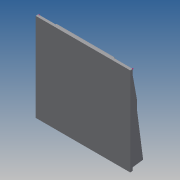
# Autodesk Inventor part: Bottom
Saved by Autodesk Inventor 2019 (Build 230136000, 136)
## iProperties
Created: 2022-10-28
Part Number: Bottom
Material: Generisch
Document SubType Name: Modeling
Designer: Dominik Schmidt
Density: 1 g/cm^3
Appearance: Vorgabe
Author: Dominik Schmidt
Autodesk Inventor part; units mm, degrees
ref_plane "YZ Plane" through (0, 0, 0) normal (1, 0, 0) x (0, 1, 0)
ref_plane "XZ Plane" through (0, 0, 0) normal (0, 1, 0) x (-1, 0, 0)
ref_plane "XY Plane" through (0, 0, 0) normal (0, 0, 1) x (1, 0, 0)
sketch "Skizze1" plane through (0, 0, 0) normal (0, 0, 1) x (1, 0, 0)
  line L0 (0, 0) -> (0, -76.0602) projected
  line L1 (0, -76.0602) -> (-35.95, -76.0602) projected
  line L2 (-45.45, -76.0602) -> (-81.4, -76.0602) projected
  line L3 (-81.4, -76.0602) -> (-81.4, 0) projected
  line L4 (-81.4, 0) -> (0, 0) projected
  line L5 (0, -76.0602) -> (-81.4, -76.0602)
  line L6 (-81.4, -76.0602) -> (-81.4, 0)
  line L7 (-81.4, 0) -> (0, 0)
  line L8 (0, 0) -> (0, -76.0602)
  constraints: 8 end point, 2 parallel, 1 horizontal, 1 perpendicular
extrude "Extrusion1" add sketch "Skizze1" along normal blind 2
sketch "Skizze2" plane through (0, 0, 0) normal (0, 0, -1) x (-1, 0, 0)
  point P0 (0, 0)
sketch "Skizze3" plane through (0, 0, 0) normal (0, 0, -1) x (-1, 0, 0)
  line L0 (35.95, -74.8497) -> (1.2, -74.8497) projected
  line L1 (80.2, -74.8497) -> (45.45, -74.8497) projected
  line L2 (49.95, -74.8497) -> (31.45, -74.8497)
  line L3 (31.45, -74.8497) -> (31.45, -50.3497)
  line L4 (31.45, -50.3497) -> (49.95, -50.3497)
  line L5 (49.95, -50.3497) -> (49.95, -74.8497)
  line L6 (81.4, 0) -> (81.4, -76.0602) projected
  line L7 (31.45, -50.3497) -> (29.45, -50.3497)
  line L8 (29.45, -50.3497) -> (29.45, -53.3497)
  line L9 (29.45, -53.3497) -> (31.45, -53.3497)
  line L10 (31.45, -53.3497) -> (31.45, -50.3497)
  line L11 (49.95, -50.3497) -> (51.95, -50.3497)
  line L12 (51.95, -50.3497) -> (51.95, -53.3497)
  line L13 (51.95, -53.3497) -> (49.95, -53.3497)
  line L14 (49.95, -53.3497) -> (49.95, -50.3497)
  line L15 (31.45, -50.3497) -> (34.45, -50.3497)
  line L16 (34.45, -50.3497) -> (34.45, -48.3497)
  line L17 (34.45, -48.3497) -> (31.45, -48.3497)
  line L18 (31.45, -48.3497) -> (31.45, -50.3497)
  line L19 (49.95, -50.3497) -> (46.95, -50.3497)
  line L20 (46.95, -50.3497) -> (46.95, -48.3497)
  line L21 (46.95, -48.3497) -> (49.95, -48.3497)
  line L22 (49.95, -48.3497) -> (49.95, -50.3497)
  line L23 (51.95, -50.3497) -> (49.95, -50.3497)
  line L24 (49.95, -50.3497) -> (49.95, -48.3497)
  line L25 (49.95, -48.3497) -> (51.95, -48.3497)
  line L26 (51.95, -48.3497) -> (51.95, -50.3497)
  line L27 (31.45, -50.3497) -> (29.45, -50.3497)
  line L28 (29.45, -50.3497) -> (29.45, -48.3497)
  line L29 (29.45, -48.3497) -> (31.45, -48.3497)
  line L30 (31.45, -48.3497) -> (31.45, -50.3497)
  point P0 (0, 0)
  dimension "d2" = 18.5
  dimension "d3" = 24.5
  dimension "d4" = 31.45
  dimension "d5" = 2
  dimension "d6" = 3
  dimension "d7" = 2
  dimension "d8" = 3
  dimension "d9" = 3
  dimension "d10" = 2
  dimension "d11" = 3
  dimension "d12" = 2
  constraints: 56 end point, 14 parallel, 7 horizontal, 7 perpendicular, 2 point on line
  measures "d2" distance of L3.end L4.end
  measures "d3" distance of L2.end L3.end
  measures "d4" distance between parallel lines of L6 L5
  measures "d5" distance of L9.end L8.end
  measures "d6" distance of L8.end L7.end
  measures "d7" distance of L12.end L13.end
  measures "d8" distance of L11.end L12.end
  measures "d9" distance of L17.end L16.end
  measures "d10" distance of L16.end L15.end
  measures "d11" distance of L20.end L21.end
  measures "d12" distance of L19.end L20.end
extrude "Extrusion2" add sketch "Skizze3" along normal blind 5 contours L9 L8 L7 L3 | L18 L17 L16 L4 | L7 L28 L29 L18 | L5 L11 L12 L13 | L22 L25 L26 L11 | L4 L20 L21 L22
sketch "Skizze4" plane through (-29.45, -53.3497, 0) normal (1, 0, 0) x (0, 0, -1)
  line L0 (9.1283, -19.2806) -> (0.7139, 44.1639) projected
  line L1 (0, -22.7105) -> (0, 53.3497) projected
  line L2 (5.629, 7.1044) -> (6.7525, -1.3669)
  line L3 (6.7525, -1.3669) -> (5.2084, -1.5716)
  line L4 (5.2084, -1.5716) -> (4.0849, 6.8996)
  line L5 (4.0849, 6.8996) -> (5.629, 7.1044)
  line L6 (5.629, 7.1044) -> (6.7525, -1.3669)
  line L7 (6.7525, -1.3669) -> (5.2084, -1.5716)
  line L8 (5.2084, -1.5716) -> (4.0849, 6.8996)
  line L9 (4.0849, 6.8996) -> (5.629, 7.1044)
  line L10 (5.629, 7.1044) -> (6.7525, -1.3669)
  line L11 (6.7525, -1.3669) -> (4.7916, -1.6269)
  line L12 (4.7916, -1.6269) -> (3.6681, 6.8444)
  line L13 (3.6681, 6.8444) -> (5.629, 7.1044)
  dimension "d17" = 1.978
  constraints: 24 end point, 6 parallel, 3 perpendicular, 2 collinear, 2 point on line
  measures "d17" distance of L2.end L11.end
extrude "Extrusion4" cut sketch "Skizze4" against normal blind 38.25
sketch "Skizze5" plane through (-51.95, -53.3497, 0) normal (-1, 0, 0) x (0, 0, 1)
  line L0 (-3.9127, 5) -> (-4.5759, 0) projected
  line L1 (0, 0) -> (-4.5759, 0) projected
  line L2 (0, 5) -> (0, 0) projected
  line L3 (0, 5) -> (-3.9127, 5) projected
  point P0 (0, 53.3497)
extrude "Extrusion5" add sketch "Skizze5" along normal blind 20
sketch "Skizze6" plane through (-71.95, -53.3497, 0) normal (-1, 0, 0) x (0, 0, 1)
  line L0 (-6.4924, -14.4505) -> (-0.5768, 30.1527)
  line L1 (-4.5759, 0) -> (-4.178, 3) projected
  line L2 (-0.5768, 30.1527) -> (0, 30.0762)
  line L3 (0, -22.7105) -> (0, 53.3497) projected
  line L4 (-6.4924, -14.4505) -> (0, -14.4505)
  line L5 (-5.5539, -7.3746) -> (0, -7.3746)
  line L6 (0, -14.4505) -> (0, -7.3746)
  line L7 (-2.5606, 15.1951) -> (0, 15.1951)
  line L8 (0, 15.1951) -> (0, 30.0762)
  constraints: 14 end point, 6 point on line, 4 perpendicular, 1 collinear, 1 horizontal, 1 parallel
extrude "Extrusion6" add sketch "Skizze6" against normal up to surface (42.5 mm away) contours L0 L5 L3 L4 | L7 L0 L2 L3
sketch "Skizze8" plane through (0, 0, 0) normal (0, 0, -1) x (-1, 0, 0)
  line L0 (34.45, -50.3497) -> (31.45, -50.3497) projected
  line L1 (71.95, -67.8002) -> (29.45, -67.8002) projected
  line L2 (31.45, -50.3497) -> (49.95, -50.3497)
  line L3 (49.95, -50.3497) -> (49.95, -67.8002)
  line L4 (49.95, -67.8002) -> (31.45, -67.8002)
  line L5 (31.45, -67.8002) -> (31.45, -50.3497)
  point P0 (0, 0)
  dimension "d24" = 18.5
  constraints: 8 end point, 2 parallel, 1 horizontal, 1 perpendicular, 1 point on line
  measures "d24" distance of L3.end L4.end
sketch "Skizze9" plane through (0, 0, 0) normal (0, 0, -1) x (-1, 0, 0)
  line L0 (56.3907, -39.4363) -> (48.4184, -39.4363)
  line L1 (48.4184, -39.4363) -> (48.4184, -20.1965)
  line L2 (48.4184, -20.1965) -> (56.3907, -20.1965)
  line L3 (56.3907, -20.1965) -> (56.3907, -39.4363)
  point P0 (0, 0)
  constraints: 8 end point, 2 parallel, 1 horizontal, 1 perpendicular
extrude "Extrusion7" cut sketch "Skizze9" along normal blind 3
extrude "Extrusion8" cut sketch "Skizze8" along normal blind 7.25
sketch "Skizze10" plane through (0, 0, 0) normal (0, 0, -1) x (-1, 0, 0)
  line L0 (80.2, -1.2105) -> (80.2, -74.8497) projected
  line L1 (1.2, -74.8497) -> (1.2, -1.2105) projected
  line L2 (80.2, -70.6388) -> (78.2, -70.6388)
  line L3 (78.2, -70.6388) -> (78.2, -6.3136)
  line L4 (78.2, -6.3136) -> (80.2, -6.3136)
  line L5 (80.2, -6.3136) -> (80.2, -70.6388)
  line L6 (1.2, -70.6388) -> (3.2, -70.6388)
  line L7 (3.2, -70.6388) -> (3.2, -6.3136)
  line L8 (3.2, -6.3136) -> (1.2, -6.3136)
  line L9 (1.2, -6.3136) -> (1.2, -70.6388)
  point P0 (0, 0)
  dimension "d29" = 2
  dimension "d30" = 2
  constraints: 16 end point, 4 parallel, 4 point on line, 2 horizontal, 2 perpendicular
  measures "d29" distance of L3.end L4.end
  measures "d30" distance of L8.end L7.end
extrude "Extrusion9" add sketch "Skizze10" along normal blind 5
sketch "Skizze11" plane through (-1.2, -70.6388, 0) normal (1, 0, 0) x (0, 0, -1)
  line L0 (0, 64.3252) -> (5, 64.3252) projected
  line L1 (1.3339, 64.3252) -> (5, 44.187)
  line L2 (5, 0) -> (5, 64.3252) projected
  line L3 (5, 64.3252) -> (1.3339, 64.3252)
  line L4 (5, 0) -> (5, 64.3252) projected
  line L5 (5, 44.187) -> (5, 64.3252)
  point P0 (0, 70.6388)
  constraints: 6 end point, 2 point on line, 1 horizontal, 1 vertical
extrude "Extrusion10" cut sketch "Skizze11" against normal blind 79
sketch "Skizze12" plane through (0, 0, 0) normal (0, 0, -1) x (-1, 0, 0)
  line L0 (1.2, -1.2105) -> (80.2, -1.2105) projected
  line L1 (67.4335, -1.2105) -> (17.4335, -1.2105)
  line L2 (17.4335, -1.2105) -> (17.4335, -3.2105)
  line L3 (17.4335, -3.2105) -> (67.4335, -3.2105)
  line L4 (67.4335, -3.2105) -> (67.4335, -1.2105)
  point P0 (0, 0)
  dimension "d35" = 50
  dimension "d36" = 2
  constraints: 8 end point, 2 parallel, 1 horizontal, 1 perpendicular, 1 point on line
  measures "d35" distance of L3.end L2.end
  measures "d36" distance of L2.end L1.end
extrude "Extrusion11" add sketch "Skizze12" along normal blind 2
sketch "Skizze13" plane through (0, -76.0602, 0) normal (1, 0, 0) x (0, 0, -1)
  line L0 (0, 76.0602) -> (5.9479, 76.8491) projected
  line L1 (0, 76.0602) -> (-2, 76.0602) projected
  line L2 (0, 76.0602) -> (-5.2711, 75.38)
  line L3 (-5.2711, 75.38) -> (-3.7519, 78.1316)
  line L4 (-3.7519, 78.1316) -> (0, 76.0602)
  constraints: 6 end point, 1 perpendicular
extrude "Extrusion12" cut sketch "Skizze13" against normal up to surface (81.4 mm away)
sketch "Skizze14" plane through (0, -76.0602, 2) normal (1, 0, 0) x (0, 0, -1)
  line L0 (17.8611, 2.1036) -> (2, 0) projected
  line L1 (2, 0) -> (0, 0) projected
  line L2 (2, 0) -> (0, -0.2653)
  line L3 (0, -0.2653) -> (0, 0)
  line L4 (0, 0) -> (2, 0)
  point P0 (2, 76.0602)
  constraints: 6 end point, 2 perpendicular
extrude "Extrusion13" add sketch "Skizze14" against normal up to surface (81.4 mm away)
sketch "Skizze15" plane through (-1.2, -70.6388, 0) normal (1, 0, 0) x (0, 0, -1)
  line L0 (13.225, -2.4569) -> (3.6274, 69.9094) projected
  line L1 (1.3339, 64.3252) -> (5, 44.187) projected
  line L2 (1.3339, 64.3252) -> (10.004, -1.0469)
  line L3 (10.004, -1.0469) -> (0, -1.0469)
  line L4 (0, -1.0469) -> (0, 64.3252)
  line L5 (0, 64.3252) -> (1.3339, 64.3252)
  point P0 (0, 70.6388)
  constraints: 8 end point, 2 perpendicular, 1 horizontal, 1 parallel
extrude "Extrusion14" add sketch "Skizze15" against normal up to surface (2 mm away)
sketch "Skizze16" plane through (-80.2, -70.6388, 0) normal (-1, 0, 0) x (0, 0, 1)
  line L0 (0, -1.0469) -> (-10.004, -1.0469) projected
  line L1 (-10.004, -1.0469) -> (-5, 36.6831) projected
  line L2 (0, 64.3252) -> (0, -1.0469) projected
  line L3 (0, 64.3252) -> (-1.3339, 64.3252) projected
  line L4 (-5, 44.187) -> (-5, 0) projected
  line L5 (-5, 36.0546) -> (-1.3339, 64.3252)
  point P0 (0, 70.6388)
  constraints: 2 end point, 2 point on line
extrude "Extrusion15" add sketch "Skizze16" against normal up to surface (2 mm away)
sketch "Skizze17" plane through (-1.2, -71.6857, 0) normal (1, 0, 0) x (0, 0, -1)
  line L0 (13.225, -1.41) -> (0, -3.164) projected
  line L1 (10.004, 0) -> (0, 0) projected
  line L2 (10.004, 0) -> (10.004, -1.8372)
  line L3 (0, 0) -> (0, -3.164)
  line L4 (0, -4.3745) -> (0, 71.6857) projected
  constraints: 4 end point, 1 collinear, 1 point on line, 1 vertical
extrude "Extrusion16" add sketch "Skizze17" against normal blind 4.75
sketch "Skizze18" plane through (-80.2, -71.6857, -10.004) normal (-1, 0, 0) x (0, 0, 1)
  line L0 (0, -1.8372) -> (10.004, -3.164) projected
  line L1 (10.004, 0) -> (10.004, -3.164) projected
  line L2 (10.004, 0) -> (0, 0) projected
  line L3 (0, 0) -> (0, -1.8372) projected
  line L4 (10.004, 0) -> (0, 0) projected
  line L5 (2.1645, 0) -> (2.1645, -2.1243)
  point P0 (10.004, 71.6857)
  constraints: 2 end point, 2 point on line, 1 perpendicular
extrude "Extrusion17" add sketch "Skizze18" against normal blind 27.25 contours L5 L2 L1 L0
fillet "Rundung2" radius 2 1 edges at (-79.2, -71.6857, -10.004)
fillet "Rundung3" radius 40 4 edges at (-2.2, -26.4519, -5) (-2.2, -33.9557, -5) (-79.2, -33.9557, -5) (-79.2, -26.4519, -5)
sketch "Skizze19" plane through (-17.4335, -3.2105, 0) normal (1, 0, 0) x (0, 0, -1)
  line L0 (0, 0) -> (0, 2) projected
  line L1 (0, 0) -> (2, 0) projected
  line L2 (2, 2) -> (2, 0) projected
  line L3 (0, 2) -> (2, 2) projected
  point P0 (0, 3.2105)
extrude "Extrusion18" add sketch "Skizze19" along normal up to surface (16.2335 mm away)
sketch "Skizze20" plane through (-67.4335, -3.2105, 0) normal (-1, 0, 0) x (0, 0, 1)
  line L0 (0, 2) -> (0, 0) projected
  line L1 (0, 2) -> (-2, 2) projected
  line L2 (-2, 0) -> (-2, 2) projected
  line L3 (0, 0) -> (-2, 0) projected
  point P0 (0, 3.2105)
extrude "Extrusion19" add sketch "Skizze20" along normal up to surface (12.7665 mm away)
